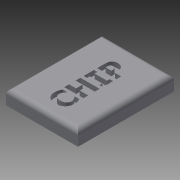
# Autodesk Inventor part: CHIP
Saved by Autodesk Inventor 2013 (Build 170138000, 138)
## iProperties
Created: 2014-07-07
Part Number: CHIP
Material: Genérico
Document SubType Name: Chapa
Designer: Administrador
Density: 1 g/cm^3
Sheet Metal Rule: Por defecto_mm
Author: Administrador
Autodesk Inventor part; units mm, degrees
note: some values were not read from the file. Chosen so that the rebuilt part matches the saved one: direction of "Repujado1".
ref_plane "YZ Plane" through (0, 0, 0) normal (1, 0, 0) x (0, 1, 0)
ref_plane "XZ Plane" through (0, 0, 0) normal (0, 1, 0) x (-1, 0, 0)
ref_plane "XY Plane" through (0, 0, 0) normal (0, 0, 1) x (1, 0, 0)
sketch "Boceto1" plane through (0, 0, 0) normal (0, 0, 1) x (1, 0, 0)
  line L0 (0, 0) -> (15, 0)
  line L1 (15, 0) -> (15, -20)
  line L2 (15, -20) -> (0, -20)
  line L3 (0, -20) -> (0, 0)
  dimension "d0" = 15
  dimension "d1" = 20
  constraints: 8 end point, 2 parallel, 1 horizontal, 1 perpendicular
  measures "d0" distance of L1.end L2.end
  measures "d1" distance of L0.end L1.end
extrude "Extrusión1" add sketch "Boceto1" along normal blind 3
sketch "Boceto2" plane through (0, 0, 3) normal (0, 0, 1) x (1, 0, 0)
  line L0 (5.7238, -17.7506) -> (5.7238, -3.3259) construction
  line L1 (5.7238, -3.3259) -> (10.4603, -3.3259) construction
  line L2 (10.4603, -3.3259) -> (10.4603, -17.7506) construction
  line L3 (10.4603, -17.7506) -> (5.7238, -17.7506) construction
  spline S0 degree 2 poles (9.8794, -15.6112) (9.8794, -16.5123) (8.7903, -17.5691) (7.8049, -17.5691) knots 0 0 0 1 2 2 2
  spline S1 degree 2 poles (7.8049, -17.5691) (6.8551, -17.5691) (5.7238, -16.5091) (5.7238, -15.608) knots 0 0 0 1 2 2 2
  spline S2 degree 2 poles (5.7238, -15.608) (5.7238, -15.3713) (5.7789, -14.9888) (5.8243, -14.8138) knots 0 0 0 1 2 2 2
  spline S3 degree 2 poles (5.8243, -14.8138) (5.8664, -14.6777) (6.0058, -14.3567) (6.0577, -14.2563) knots 0 0 0 1 2 2 2
  line L4 (6.0577, -14.2563) -> (7.0107, -14.2563)
  line L5 (7.0107, -14.2563) -> (7.0107, -14.3567)
  spline S4 degree 2 poles (7.0107, -14.3567) (6.9459, -14.4313) (6.7643, -14.6517) (6.6801, -14.7911) knots 0 0 0 1 2 2 2
  spline S5 degree 2 poles (6.6801, -14.7911) (6.5925, -14.9305) (6.4726, -15.2644) (6.4726, -15.4491) knots 0 0 0 1 2 2 2
  spline S6 degree 2 poles (6.4726, -15.4491) (6.4726, -15.6663) (6.6088, -16.0261) (6.7806, -16.1914) knots 0 0 0 1 2 2 2
  spline S7 degree 2 poles (6.7806, -16.1914) (6.9329, -16.3405) (7.4548, -16.5318) (7.8081, -16.5318) knots 0 0 0 1 2 2 2
  spline S8 degree 2 poles (7.8081, -16.5318) (8.1809, -16.5318) (8.6898, -16.3341) (8.8454, -16.172) knots 0 0 0 1 2 2 2
  spline S9 degree 2 poles (8.8454, -16.172) (8.9977, -16.0164) (9.1306, -15.6339) (9.1306, -15.4426) knots 0 0 0 1 2 2 2
  spline S10 degree 2 poles (9.1306, -15.4426) (9.1306, -15.2449) (8.9977, -14.8851) (8.9167, -14.7619) knots 0 0 0 1 2 2 2
  spline S11 degree 2 poles (8.9167, -14.7619) (8.8357, -14.6258) (8.6639, -14.4216) (8.5958, -14.347) knots 0 0 0 1 2 2 2
  line L6 (8.5958, -14.347) -> (8.5958, -14.2563)
  line L7 (8.5958, -14.2563) -> (9.5358, -14.2563)
  spline S12 degree 2 poles (9.5358, -14.2563) (9.5877, -14.3665) (9.7173, -14.655) (9.7627, -14.8106) knots 0 0 0 1 2 2 2
  spline S13 degree 2 poles (9.7627, -14.8106) (9.8211, -14.9986) (9.8794, -15.3259) (9.8794, -15.6112) knots 0 0 0 1 2 2 2
  line L8 (9.8016, -10.2887) -> (9.8016, -11.2935)
  line L9 (9.8016, -11.2935) -> (8.0285, -11.2935)
  line L10 (8.0285, -11.2935) -> (8.0285, -12.6582)
  line L11 (8.0285, -12.6582) -> (9.8016, -12.6582)
  line L12 (9.8016, -12.6582) -> (9.8016, -13.6631)
  line L13 (9.8016, -13.6631) -> (5.8016, -13.6631)
  line L14 (5.8016, -13.6631) -> (5.8016, -12.6582)
  line L15 (5.8016, -12.6582) -> (7.2668, -12.6582)
  line L16 (7.2668, -12.6582) -> (7.2668, -11.2935)
  line L17 (7.2668, -11.2935) -> (5.8016, -11.2935)
  line L18 (5.8016, -11.2935) -> (5.8016, -10.2887)
  line L19 (5.8016, -10.2887) -> (9.8016, -10.2887)
  line L20 (9.8016, -7.4686) -> (9.8016, -9.6209)
  line L21 (9.8016, -9.6209) -> (9.1047, -9.6209)
  line L22 (9.1047, -9.6209) -> (9.1047, -9.0472)
  line L23 (9.1047, -9.0472) -> (6.4985, -9.0472)
  line L24 (6.4985, -9.0472) -> (6.4985, -9.6209)
  line L25 (6.4985, -9.6209) -> (5.8016, -9.6209)
  line L26 (5.8016, -9.6209) -> (5.8016, -7.4686)
  line L27 (5.8016, -7.4686) -> (6.4985, -7.4686)
  line L28 (6.4985, -7.4686) -> (6.4985, -8.0423)
  line L29 (6.4985, -8.0423) -> (9.1047, -8.0423)
  line L30 (9.1047, -8.0423) -> (9.1047, -7.4686)
  line L31 (9.1047, -7.4686) -> (9.8016, -7.4686)
  spline S14 degree 2 poles (7.0626, -3.7247) (7.3413, -3.7247) (7.847, -3.9029) (8.0156, -4.0683) knots 0 0 0 1 2 2 2
  spline S15 degree 2 poles (8.0156, -4.0683) (8.1225, -4.1687) (8.2976, -4.4151) (8.3592, -4.561) knots 0 0 0 1 2 2 2
  spline S16 degree 2 poles (8.3592, -4.561) (8.4207, -4.7101) (8.4921, -5.0569) (8.4921, -5.2708) knots 0 0 0 1 2 2 2
  line L32 (8.4921, -5.2708) -> (8.4921, -5.796)
  line L33 (8.4921, -5.796) -> (9.8016, -5.796)
  line L34 (9.8016, -5.796) -> (9.8016, -6.8008)
  line L35 (9.8016, -6.8008) -> (5.8016, -6.8008)
  line L36 (5.8016, -6.8008) -> (5.8016, -5.2482)
  spline S17 degree 2 poles (5.8016, -5.2482) (5.8016, -4.9046) (5.928, -4.4021) (6.0642, -4.1979) knots 0 0 0 1 2 2 2
  spline S18 degree 2 poles (6.0642, -4.1979) (6.2165, -3.971) (6.7157, -3.7247) (7.0626, -3.7247) knots 0 0 0 1 2 2 2
  spline S19 degree 2 poles (7.0885, -4.7554) (6.9167, -4.7554) (6.6736, -4.9175) (6.6282, -5.0277) knots 0 0 0 1 2 2 2
  spline S20 degree 2 poles (6.6282, -5.0277) (6.5666, -5.1704) (6.5472, -5.4297) (6.5472, -5.6533) knots 0 0 0 1 2 2 2
  line L37 (6.5472, -5.6533) -> (6.5472, -5.796)
  line L38 (6.5472, -5.796) -> (7.7465, -5.796)
  line L39 (7.7465, -5.796) -> (7.7465, -5.7247)
  spline S21 degree 2 poles (7.7465, -5.7247) (7.7465, -5.5853) (7.74, -5.3324) (7.7238, -5.2384) knots 0 0 0 1 2 2 2
  spline S22 degree 2 poles (7.7238, -5.2384) (7.7109, -5.1574) (7.6331, -4.9791) (7.5844, -4.9305) knots 0 0 0 1 2 2 2
  spline S23 degree 2 poles (7.5844, -4.9305) (7.4872, -4.8268) (7.27, -4.7554) (7.0885, -4.7554) knots 0 0 0 1 2 2 2
  constraints: 2 other
emboss "Repujado1" sketch "Boceto2" operation cut depth 1 direction (0, 0, -1)
fillet "Empalme1" radius 1 4 edges at (7.5, 0, 3) (0, -10, 3) (15, -10, 3) (7.5, -20, 3)
equation "\"Radio_pliegue\" = Grosor"
equation "\"Anchura_desahogo_plegado\" = Grosor"
equation "\"Profundidad_desahogo_plegado\" = 0.5 * Grosor"
equation "\"Tamaño_destalonado\" = 4 * Grosor"
equation "\"Remanente_mínimo\" = 2 * Grosor"
equation "\"Radiodetransición\" = Radio_pliegue"
equation "\"Tamaño_de_radio_de_Jacobi\" = Radio_pliegue"
equation "\"TamañoSeparación\" = Grosor"
equation "\"Grosor\" = 0.5"
